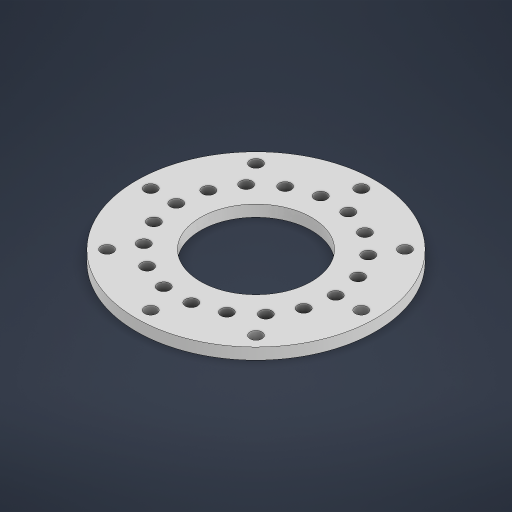
# Autodesk Inventor part: HousingExampleLid
Saved by Autodesk Inventor 2024 (Build 280153000, 153)
## iProperties
Created: 2024-03-11
Part Number: HousingExampleLid
Material: Generic
Document SubType Name: Modeling
Designer: avsar
Density: 1 g/cm^3
Appearance: Default
Author: avsar
Autodesk Inventor part; units mm, degrees
ref_plane "YZ Plane" through (0, 0, 0) normal (1, 0, 0) x (0, 1, 0)
ref_plane "XZ Plane" through (0, 0, 0) normal (0, 1, 0) x (-1, 0, 0)
ref_plane "XY Plane" through (0, 0, 0) normal (0, 0, 1) x (1, 0, 0)
sketch "Sketch1" plane through (0, 0, 0) normal (0, 1, 0) x (-1, 0, 0)
  circle A0 centre (0, 0) radius 42
  circle A1 centre (0, 0) radius 19.5
  circle A2 centre (0, -37) radius 2.1
  circle A3 centre (26.163, -26.163) radius 2.1
  circle A4 centre (37, 0) radius 2.1
  circle A5 centre (26.163, 26.163) radius 2.1
  circle A6 centre (0, 37) radius 2.1
  circle A7 centre (-26.163, 26.163) radius 2.1
  circle A8 centre (-37, 0) radius 2.1
  circle A9 centre (-26.163, -26.163) radius 2.1
  circle A10 centre (-4.8621, -27.5746) radius 2.1
  circle A11 centre (4.8621, -27.5746) radius 2.1
  circle A12 centre (14, -24.2487) radius 2.1
  circle A13 centre (21.4492, -17.9981) radius 2.1
  circle A14 centre (26.3114, -9.5766) radius 2.1
  circle A15 centre (28, 0) radius 2.1
  circle A16 centre (26.3114, 9.5766) radius 2.1
  circle A17 centre (21.4492, 17.9981) radius 2.1
  circle A18 centre (14, 24.2487) radius 2.1
  circle A19 centre (4.8621, 27.5746) radius 2.1
  circle A20 centre (-4.8621, 27.5746) radius 2.1
  circle A21 centre (-14, 24.2487) radius 2.1
  circle A22 centre (-21.4492, 17.9981) radius 2.1
  circle A23 centre (-26.3114, 9.5766) radius 2.1
  circle A24 centre (-28, 0) radius 2.1
  circle A25 centre (-26.3114, -9.5766) radius 2.1
  circle A26 centre (-21.4492, -17.9981) radius 2.1
  circle A27 centre (-14, -24.2487) radius 2.1
  line L0 (0, 0) -> (-4.8621, -27.5746) construction
  line L1 (0, 0) -> (0, -11.0753) construction
  dimension "d2" = 84
  dimension "d3" = 39
  dimension "d4" = 4.2
  dimension "d5" = 37
  dimension "d6" = 360
  dimension "d9" = 4.2
  dimension "d10" = 28
  dimension "d11" = 360
  dimension "d12" = 10
  constraints: 28 centre point, 5 coincident, 4 end point, 1 vertical, 1 vertical alignment, 54 other
  measures "d2" diameter of A0
  measures "d3" diameter of A1
  measures "d4" diameter of A2
  measures "d5" distance of A2.centre point (0, 0)
  measures "d9" diameter of A10
  measures "d10" distance of L0.start A10.centre
  measures "d12" angle of L1 L0
extrude "Extrusion1" add sketch "Sketch1" along normal blind 4
body "Solid1"
